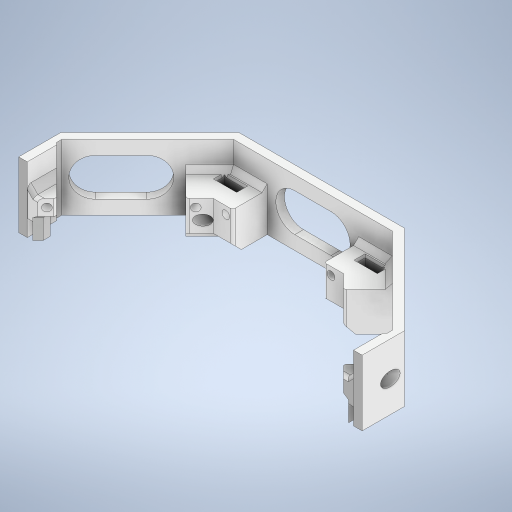
# Autodesk Inventor part: Držák TF-Luna
Saved by Autodesk Inventor 2024 (Build 280153000, 153)
## iProperties
Created: 2023-11-02
Part Number: Držák TF-Luna
Material: Všeobecné
Document SubType Name: Modeling
Designer: 42060
Density: 1 g/cm^3
Appearance: Výchozí
Author: 42060
Autodesk Inventor part; units mm, degrees
ref_plane "YZ Plane" through (0, 0, 0) normal (1, 0, 0) x (0, 1, 0)
ref_plane "XZ Plane" through (0, 0, 0) normal (0, 1, 0) x (-1, 0, 0)
ref_plane "XY Plane" through (0, 0, 0) normal (0, 0, 1) x (1, 0, 0)
sketch "Náčrt1" plane through (0, 0, 0) normal (0, 0, 1) x (1, 0, 0)
  line L0 (0, 0) -> (0, -2.5)
  line L1 (0, -2.5) -> (23, -2.5)
  line L2 (23, -2.5) -> (47.25, -26.75)
  line L3 (49.75, -25.7145) -> (24.0355, 0)
  line L4 (24.0355, 0) -> (0, 0)
  line L5 (49.75, -25.7145) -> (49.75, -37.923)
  line L6 (49.75, -37.923) -> (47.25, -37.923)
  line L7 (47.25, -37.923) -> (47.25, -26.75)
  dimension "d0" = 2.5
  dimension "d1" = 23
  dimension "d2" = 135
  dimension "d50" = 49.75
  dimension "d54" = 2.5
  dimension "d55" = 2.5
  dimension "d156" = 37.923
  constraints: 16 end point, 3 perpendicular, 2 vertical, 1 parallel
  measures "d0" distance of L0.start L0.end
  measures "d1" distance of L0.end L1.end
  measures "d2" angle of L2 L1
  measures "d50" distance between parallel lines of L5 L0
  measures "d54" distance between parallel lines of L2 L3
  measures "d55" distance between parallel lines of L5 L7
  measures "d156" distance between parallel lines of L6 L4
extrude "Vysunutí1" add sketch "Náčrt1" along normal mid plane 19
sketch "Náčrt2" plane through (0, -2.5, 9.5) normal (0, -1, 0) x (1, 0, 0)
  line L0 (23, -19) -> (23, 0) projected
  line L1 (0, 0) -> (23, 0) projected
  line L2 (0, -19) -> (0, 0) projected
  line L3 (23, -19) -> (0, -19) projected
  line L4 (13.25, -7.75) -> (15.25, -7.75)
  arc A0 (15.25, -12.25) -> (15.25, -7.75) centre (15.25, -10) ccw
  line L5 (15.25, -12.25) -> (13.25, -12.25)
  line L6 (13.25, -12.25) -> (13.25, -7.75)
  point P0 (0, -9.5)
  dimension "d6" = 2.25
  dimension "d8" = 9
  dimension "d148" = 13.25
  dimension "d149" = 15.25
  constraints: 6 end point, 2 point on circle, 2 tangent, 1 centre point, 1 horizontal, 1 parallel, 1 perpendicular
  measures "d6" radius of A0
  measures "d8" distance from line of L3 A0.centre
  measures "d148" distance between parallel lines of L6 L2
  measures "d149" distance from line of L2 A0.centre
extrude "Vysunutí2" add sketch "Náčrt2" along normal blind 10 contours L4 A0 L5 L6
sketch "Náčrt4" plane through (47.25, -26.75, 9.5) normal (-0.7071068, -0.7071068, 0) x (-0.7071068, 0.7071068, 0)
  line L0 (24.5447, 7.75) -> (26.5447, 7.75)
  arc A0 (26.5447, 7.75) -> (26.5447, 12.25) centre (26.5447, 10) ccw
  line L1 (26.5447, 12.25) -> (24.5447, 12.25)
  line L2 (24.5447, 12.25) -> (24.5447, 7.75)
  line L3 (0, 19) -> (0, 0) projected
  line L4 (34.2947, 0) -> (0, 0) projected
  line L5 (34.2947, 19) -> (34.2947, 0) projected
  line L6 (0, 19) -> (34.2947, 19) projected
  line L7 (41.189, 12.25) -> (41.189, 7.75) projected
  line L8 (11.2947, 19) -> (11.2947, 0) construction
  line L9 (-1.9553, 12.25) -> (-1.9553, 7.75)
  line L10 (-1.9553, 7.75) -> (-6.4553, 7.75)
  line L11 (-6.4553, 7.75) -> (-6.4553, 12.25)
  line L12 (-6.4553, 12.25) -> (-1.9553, 12.25)
  point P0 (52.3259, 9.5)
  point P1 (28.7947, 10)
  point P2 (-3.9553, 10)
  dimension "d22" = 15.25
  dimension "d33" = 2.25
  dimension "d39" = 5.5
  dimension "d150" = 13.25
  constraints: 16 end point, 4 perpendicular, 3 point on circle, 3 symmetric about line, 2 horizontal, 2 point on line, 2 tangent, 1 centre point, 1 horizontal alignment, 1 parallel, 1 vertical
  measures "d22" distance from line of L8 A0.centre
  measures "d33" radius of A0
  measures "d39" distance from line of L5 point (28.795, 10)
  measures "d150" distance between parallel lines of L8 L2
extrude "Vysunutí3" add sketch "Náčrt4" along normal blind 10 contours L2 L1 A0 L0 | L9 L10 L11 L12
sketch "Náčrt8" plane through (49.75, -37.923, 9.5) normal (1, 0, 0) x (0, 0, -1)
  line L0 (7.75, 8.673) -> (12.25, 8.673) projected
  line L1 (7.75, 6.6084) -> (7.75, 8.673) projected
  line L2 (12.25, 6.6084) -> (7.75, 6.6084) projected
  line L3 (12.25, 8.673) -> (12.25, 6.6084) projected
  line L4 (12.25, 4.5438) -> (7.75, 4.5438) projected
  line L5 (12.25, 6.6084) -> (12.25, 4.5438) projected
  line L6 (12.25, 6.6084) -> (7.75, 6.6084) projected
  line L7 (7.75, 6.6084) -> (7.75, 4.5438) projected
  point P0 (9.5, 37.923)
extrude "Vysunutí7" cut sketch "Náčrt8" along normal through all
sketch "Náčrt10" plane through (13.25, -2.5, 1.75) normal (0, 0, 1) x (1, 0, 0)
  line L0 (2, -10) -> (0, -10) projected
  line L1 (2, -10) -> (4.25, -10) projected
  line L2 (6.568, -10.9602) -> (8.159, -12.5511) projected
  line L3 (9.5732, -13.9654) -> (8.159, -12.5511) projected
  line L4 (4.25, -10) -> (5.6079, -10)
  line L5 (5.6079, -10) -> (6.568, -10.9602)
  circle A0 centre (7.8444, -4.6004) radius 3.5944
  line L6 (4.25, 0) -> (4.25, -10) projected
  line L7 (13.6391, -3.8891) -> (6.568, -10.9602) projected
  line L8 (4.25, -4.6004) -> (2, -4.6004)
  line L9 (2, 0) -> (2, -10) projected
  line L10 (10.3861, -7.1421) -> (11.9771, -8.7331)
  line L11 (15.2301, -5.4801) -> (8.159, -12.5511) projected
  line L12 (5.6079, -10) -> (6.4689, -7.9213) construction
  line L13 (-13.25, 0) -> (9.75, 0) projected
  line L14 (9.75, 0) -> (34, -24.25) projected
  point P0 (-13.25, 2.5)
  dimension "d70" = 112.5
  constraints: 10 end point, 4 point on line, 3 point on circle, 2 horizontal, 2 tangent, 1 centre point, 1 collinear, 1 equal length, 1 perpendicular
  measures "d70" angle of L4 L12
extrude "Vysunutí9" add sketch "Náčrt10" against normal up to surface (4.5 mm away) contours L9 L8 L6 L1 | L6 A0 L7 L5 L4 | L9 L13 L6 L8 | L7 L10 L11 L2 | L7 L14 L11 L10
sketch "Náčrt6" plane through (47.25, -26.75, 9.5) normal (-0.7071068, -0.7071068, 0) x (-0.7071068, 0.7071068, 0)
  arc A0 (11.3919, 8.2595) -> (11.3919, 10.7405) centre (16.5447, 9.5) ccw
  arc A1 (11.1975, 10.7405) -> (11.1975, 8.2595) centre (6.0447, 9.5) ccw
  line L0 (0, 19) -> (0, 0) projected
  line L1 (24.5447, 12.25) -> (24.5447, 7.75) projected
  line L2 (-1.9553, 7.75) -> (-1.9553, 12.25) projected
  line L3 (16.5447, 9.5) -> (24.5447, 9.5) construction
  line L4 (6.0447, 9.5) -> (-1.9553, 9.5) construction
  arc A2 (11.3919, 8.2595) -> (11.1975, 8.2595) centre (11.2947, 8.2361) ccw
  arc A3 (11.1975, 10.7405) -> (11.3919, 10.7405) centre (11.2947, 10.7639) ccw
  arc A4 (11.2947, 7.8606) -> (11.2947, 11.1394) centre (16.5447, 9.5) ccw
  arc A5 (11.2947, 11.1394) -> (11.2947, 7.8606) centre (6.0447, 9.5) ccw
  line L5 (16.5447, 4) -> (6.0447, 4)
  line L6 (16.5447, 15) -> (6.0447, 15)
  point P0 (52.3259, 9.5)
  point P1 (12.5018, 10.2263)
  point P2 (12.5018, 8.7737)
  point P3 (0, 9.5)
  point P4 (12.599, 10.7405)
  point P5 (12.4046, 10.7405)
  point P6 (12.4046, 8.2595)
  point P7 (12.599, 8.2595)
  dimension "d44" = 10.6
  dimension "d45" = 10.5
  dimension "d48" = 0.2
  dimension "d114" = 0.2
  constraints: 16 point on circle, 8 end point, 7 tangent, 6 centre point, 3 point on line, 2 equal radius, 2 horizontal alignment, 1 collinear, 1 midpoint, 1 parallel, 1 perpendicular, 1 other
  measures "d44" diameter of A1
  measures "d45" distance of L4.start L3.start
  measures "d48" diameter of A2
  measures "d114" radial gap between concentric circles of A0 A4
extrude "Vysunutí5" cut sketch "Náčrt6" against normal blind 11.5 contours A2 A1 A3 A0 | A5 A4 | A4 L5 A5 | A4 A5 L6
sketch "Náčrt7" plane through (0, -2.5, 9.5) normal (0, -1, 0) x (1, 0, 0)
  arc A0 (0.0972, -10.7405) -> (0.0972, -8.2595) centre (5.25, -9.5) ccw
  line L0 (0, -19) -> (0, 0) projected
  arc A1 (0, -8.3361) -> (0.0972, -8.2595) centre (0, -8.2361) ccw
  arc A2 (0.0972, -10.7405) -> (0, -10.6639) centre (0, -10.7639) ccw
  arc A3 (-0.0972, -8.2595) -> (-0.0972, -10.7405) centre (-5.25, -9.5) ccw
  arc A4 (-0.0972, -8.2595) -> (0, -8.3361) centre (0, -8.2361) ccw
  arc A5 (0, -10.6639) -> (-0.0972, -10.7405) centre (0, -10.7639) ccw
  arc A6 (0, -7.8606) -> (0, -11.1394) centre (-5.25, -9.5) ccw
  arc A7 (0, -11.1394) -> (0, -7.8606) centre (5.25, -9.5) ccw
  line L1 (-5.25, -4) -> (5.25, -4)
  line L2 (-5.25, -15) -> (5.25, -15)
  point P0 (0, -9.5)
  point P1 (0, -9.5)
  point P2 (0, -8.7737)
  point P3 (0, -10.2263)
  point P4 (0, -9.5)
  point P5 (0.0972, -8.2595)
  point P6 (0, -8.3361)
  point P7 (0, -10.6639)
  point P8 (0.0972, -10.7405)
  point P9 (0, -8.1361)
  point P10 (0, -10.8639)
  point P11 (0, -11.1394)
  point P12 (0, -15)
  point P13 (0, -4)
  dimension "d40" = 10.6
  dimension "d41" = 5.25
  dimension "d49" = 0.2
  dimension "d115" = 0.2
  constraints: 20 point on circle, 8 centre point, 6 tangent, 4 end point, 3 symmetric about line, 2 midpoint, 2 point on line, 2 vertical alignment, 1 equal radius, 1 horizontal alignment, 4 other
  measures "d40" diameter of A0
  measures "d41" distance from line of A0.centre L0
  measures "d49" diameter of A1
  measures "d115" radial gap between concentric circles of A3 A6
extrude "Vysunutí4" cut sketch "Náčrt7" against normal blind 11.5 contours A2 L0 A1 A0 | A0 A1 L0 A7 A2 | A5 A3 A4 L0 | A7 L2 L0 | L0 L1 A7
sketch "Náčrt11" plane through (0, 0, -9.5) normal (0, 0, -1) x (-1, 0, 0)
  line L0 (-23, -2.5) -> (0, -2.5) projected
  line L1 (-47.25, -26.75) -> (-23, -2.5) projected
  line L2 (-13.25, -2.5) -> (-13.25, -12.5) projected
  line L3 (-13.25, -12.5) -> (-18.8579, -12.5) projected
  line L4 (-18.8579, -12.5) -> (-22.8232, -16.4654) projected
  line L5 (-29.8943, -9.3943) -> (-22.8232, -16.4654) projected
  arc A0 (-23.6361, -9.6421) -> (-17.5, -7.1004) centre (-21.0944, -7.1004) ccw projected
  line L6 (-17.5, -7.1004) -> (-17.5, -2.5) projected
  line L7 (-26.8891, -6.3891) -> (-23.6361, -9.6421) projected
  point P0 (0, 0)
extrude "Vysunutí10" add sketch "Náčrt11" against normal up to surface (6.75 mm away) contours L0 L2 L3 L4 L5 L1 L7 A0 L6
sketch "Náčrt3" plane through (0, -12.5, 9.5) normal (0, -1, 0) x (1, 0, 0)
  arc A0 (15.25, -12.25) -> (15.25, -7.75) centre (15.25, -10) ccw projected
  point P0 (0, -9.5)
  constraints: 1 coincident
hole "Díra1" at (15.25, -12.5, -0.5) direction (0, 1, 0) diameter 2.2 end through all
sketch "Náčrt5" plane through (40.1789, -33.8211, 9.5) normal (-0.7071068, -0.7071068, 0) x (0, 0, -1)
  arc A0 (7.75, -26.5447) -> (12.25, -26.5447) centre (10, -26.5447) ccw projected
  line L0 (12.25, 6.4553) -> (7.75, 6.4553) projected
  line L1 (7.75, 6.4553) -> (7.75, 1.9553) projected
  line L2 (7.75, 1.9553) -> (12.25, 1.9553) projected
  line L3 (12.25, 1.9553) -> (12.25, 6.4553) projected
  line L4 (12.25, 1.9553) -> (12.25, 6.4553) projected
  line L5 (12.25, 6.4553) -> (7.75, 6.4553) projected
  line L6 (19, 1.0355) -> (0, 1.0355) projected
  line L7 (0, 9.6683) -> (0, 1.0355) projected
  line L8 (19, 9.6683) -> (0, 9.6683) projected
  line L9 (19, 1.0355) -> (19, 9.6683) projected
  line L10 (19, -11.2947) -> (0, -11.2947) construction
  point P0 (9.5, -52.3259)
  point P1 (10, 3.9553)
  constraints: 1 coincident, 1 symmetric about line
hole "Díra2" at (21.409, -15.0511, -0.5) at (42.9758, -36.6179, -0.5) direction (0.7071068, 0.7071068, 0) diameter 2.2 end through all
chamfer "Zkosení3" [suppressed]
sketch "Náčrt9" plane through (47.25, -35.8792, 1.75) normal (0, 0, 1) x (1, 0, 0)
  line L0 (0, -2.0438) -> (0, 9.1292) projected
  line L1 (0, 0) -> (-2.5065, -2.5065) projected
  line L2 (0, -2.0438) -> (-2.0438, -2.0438)
  line L3 (-2.0438, -2.0438) -> (-2.9691, -2.0438)
  line L4 (-2.5065, -2.5065) -> (-5.6884, 0.6755) projected
  line L5 (0, 9.1292) -> (0, -2.0438) projected
  point P0 (-47.25, 35.8792)
  constraints: 4 end point, 2 horizontal, 2 point on line
extrude "Vysunutí8" add sketch "Náčrt9" against normal up to surface (4.5 mm away) contours L2 L1 L0
extrude "Vysunutí17" cut sketch "Náčrt9" against normal through all contours L1 L4 L3
sketch "Náčrt25" plane through (47.25, -35.8792, -2.75) normal (0, 0, -1) x (-1, 0, 0)
  line L0 (1.5, 2.9562) -> (1.5, -2.0438)
  line L1 (1.5, -2.0438) -> (3, -0.5438)
  line L2 (3, -0.5438) -> (3, 1.4562)
  line L3 (3, 1.4562) -> (1.5, 2.9562)
  line L4 (0, -2.0438) -> (0, 9.1292) projected
  point P0 (47.25, 35.8792)
  dimension "d185" = 45
  dimension "d188" = 1.5
  dimension "d189" = 5
  dimension "d190" = 1.5
  dimension "d191" = 45
  constraints: 8 end point, 1 horizontal alignment, 1 parallel, 1 vertical
  measures "d185" angle of L3 L0
  measures "d188" distance between parallel lines of L0 L2
  measures "d189" distance of L0.start L0.end
  measures "d190" distance between parallel lines of L4 L0
  measures "d191" angle of L0 L1
extrude "Vysunutí24" add sketch "Náčrt25" along normal up to surface (6.75 mm away)
chamfer "Zkosení4" [suppressed]
chamfer "Zkosení10" distance 2 angle 45 2 edges at (47.25, -33.7191, 1.75) (47.25, -33.7191, -2.75)
chamfer "Zkosení11" distance 1.0388 angle 45 3 edges at (44.75, -33.923, -2.75) (44.25, -35.423, -2.75) (44.75, -36.923, -2.75)
sketch "Náčrt26" plane through (47.25, -37.923, 9.5) normal (0, -1, 0) x (1, 0, 0)
  line L0 (0, -14.25) -> (-1.5, -14.25)
  line L1 (2.5, -19) -> (2.5, 0) projected
  line L2 (0, 0) -> (2.5, 0) projected
  line L3 (0, -5.75) -> (0, 0) projected
  line L4 (-2, -7.75) -> (0, -5.75) projected
  line L5 (-2.9691, -7.75) -> (-2, -7.75) projected
  line L6 (-2.9691, -12.25) -> (-2.9691, -7.75) projected
  line L7 (-2.9691, -12.25) -> (-2.9691, -12.25) projected
  line L8 (-2.9691, -12.25) -> (-1.5, -13.2888) projected
  line L9 (-1.5, -12.75) -> (-1.5, -13.2888) projected
  line L10 (0, -14.25) -> (-1.5, -12.75) projected
  line L11 (0, -19) -> (0, -14.25) projected
  line L12 (2.5, -19) -> (0, -19) projected
  line L13 (-1.5, -13.2888) -> (-1.5, -19) projected
  point P0 (-47.25, -9.5)
  constraints: 2 end point, 1 horizontal
extrude "Vysunutí25" add sketch "Náčrt26" against normal up to surface contours L0 L13 L9 L10 surface through (44.25, -34.423, -2.75) normal (-0.7071068, 0.7071068, 0)
extrude "Vysunutí21" add sketch "Náčrt11" against normal blind 2.5 contours L0 L6 A0 L7 L1
sketch "Náčrt22" plane through (17.5, -2.5, -7) normal (0, 0, 1) x (1, 0, 0)
  line L0 (0, -2.4004) -> (5.75, -2.4004)
  line L1 (5.75, -2.4004) -> (5.75, -4.6004)
  line L2 (5.75, -4.6004) -> (0, -4.6004)
  line L3 (0, -4.6004) -> (0, -2.4004)
  line L4 (0, -4.6004) -> (0, 0) projected
  arc A0 (0, -4.6004) -> (6.1361, -7.1421) centre (3.5944, -4.6004) ccw projected
  line L5 (9.3891, -3.8891) -> (6.1361, -7.1421) projected
  line L6 (5.5, 0) -> (9.3891, -3.8891) projected
  line L7 (0, 0) -> (5.5, 0) projected
  point P0 (-17.5, 2.5)
  point P1 (0, -2.4004)
  dimension "d163" = 5.75
  dimension "d164" = 2.2
  constraints: 8 end point, 2 parallel, 1 collinear, 1 horizontal, 1 perpendicular, 1 point on line
  measures "d163" distance of L1.end L2.end
  measures "d164" distance of L0.end L1.end
extrude "Vysunutí20" add sketch "Náčrt22" along normal up to surface (8.75 mm away) contours L4 L7 L6 L5 A0 L2 L1 L0
sketch "Náčrt23" plane through (17.5, -4.9004, -7) normal (0, -1, 0) x (1, 0, 0)
  line L0 (5.75, 8.75) -> (0, 8.75) projected
  line L1 (0, 0) -> (0, 8.75) projected
  line L2 (5.75, 0) -> (0, 0) projected
  line L3 (5.75, 0) -> (5.75, 8.75) projected
  line L4 (0, 1.6599) -> (2.875, 0)
  line L5 (2.875, 0) -> (5.75, 1.6599)
  circle A0 centre (2.875, 3.3198) radius 2.875 construction
  point P0 (-17.5, 7)
  dimension "d169" = 120
  constraints: 4 end point, 3 tangent, 2 point on line, 1 centre point, 1 horizontal alignment, 1 midpoint
  measures "d169" angle of L5 L4
extrude "Vysunutí22" add sketch "Náčrt23" along normal up to surface (2.2 mm away) contours L3 L2 L5 | L4 L2 L1
hole "Díra6" at (20.375, -4.9004, -3.6802) direction (0, 1, 0) diameter 3 end through all both
sketch "Náčrt24" plane through (0, 0, -9.5) normal (0, 0, -1) x (-1, 0, 0)
  line L0 (0, 0) -> (-24.0355, 0) projected
  line L1 (-17.5, -7.1004) -> (-17.5, -4.9004) projected
  line L2 (-17.5, -7.1004) -> (-17.5, -4.9004) projected
  line L3 (-21.875, 0) -> (-18.875, 0) projected
  line L4 (-18.875, -4.9004) -> (-21.875, -4.9004) projected
  line L5 (-23.25, -2) -> (-17.5, -2)
  line L6 (-23.25, -2) -> (-22.7141, 0)
  line L7 (-17.5, -2) -> (-18.0359, 0)
  point P0 (-20.375, -2)
  point P1 (-20.375, -4.9004)
  dimension "d180" = 2
  dimension "d183" = 75
  dimension "d184" = 75
  constraints: 6 end point, 3 point on line, 2 midpoint, 1 vertical alignment
  measures "d180" distance between parallel lines of L0 L5
  measures "d183" angle of L0 L6
  measures "d184" angle of L0 L7
extrude "Vysunutí23" cut sketch "Náčrt24" against normal blind 10
fillet "Zaoblení1" radius 1 2 edges at (46.25, -37.923, 2.75) (44.7654, -37.923, 1.75)
chamfer "Zkosení5" distance 1.5 angle 45 2 edges at (26.4471, -5.9471, 1.75) (18.125, -2.5, 1.75)
sketch "Náčrt12" plane through (0, 0, 9.5) normal (0, 1, 0) x (1, 0, 0)
  circle A0 centre (15.25, 10) radius 1.1 projected
  line L0 (15.25, 12.4249) -> (17.35, 11.2124)
  line L1 (17.35, 11.2124) -> (17.35, 8.7876)
  line L2 (17.35, 8.7876) -> (15.25, 7.5751)
  line L3 (15.25, 7.5751) -> (13.15, 8.7876)
  line L4 (13.15, 8.7876) -> (13.15, 11.2124)
  line L5 (13.15, 11.2124) -> (15.25, 12.4249)
  point P0 (0, 9.5)
  point P1 (15.25, 10)
  dimension "d81" = 4.2
  constraints: 12 end point, 1 coincident, 1 vertical alignment, 13 other
  measures "d81" distance between parallel lines of L4 L1
extrude "Vysunutí12" [suppressed]
sketch "Náčrt13" plane through (24.0355, 0, -9.5) normal (0.7071068, 0.7071068, 0) x (-0.7071068, 0.7071068, 0)
  circle A0 centre (-8.7855, 9) radius 1.1 projected
  line L0 (-8.7855, 6.5751) -> (-10.8855, 7.7876)
  line L1 (-10.8855, 7.7876) -> (-10.8855, 10.2124)
  line L2 (-10.8855, 10.2124) -> (-8.7855, 11.4249)
  line L3 (-8.7855, 11.4249) -> (-6.6855, 10.2124)
  line L4 (-6.6855, 10.2124) -> (-6.6855, 7.7876)
  line L5 (-6.6855, 7.7876) -> (-8.7855, 6.5751)
  line L6 (-39.2855, 6.5751) -> (-41.3855, 7.7876)
  line L7 (-41.3855, 7.7876) -> (-41.3855, 10.2124)
  line L8 (-41.3855, 10.2124) -> (-39.2855, 11.4249)
  line L9 (-39.2855, 11.4249) -> (-37.1855, 10.2124)
  line L10 (-37.1855, 10.2124) -> (-37.1855, 7.7876)
  line L11 (-37.1855, 7.7876) -> (-39.2855, 6.5751)
  circle A1 centre (-39.2855, 9) radius 1.1 projected
  point P0 (16.9957, 9.5)
  point P1 (-39.2855, 9)
  point P2 (-39.2855, 9)
  dimension "d84" = 4.2
  dimension "d85" = 4.2
  constraints: 24 end point, 3 coincident, 1 vertical alignment, 26 other
  measures "d84" distance between parallel lines of L4 L1
  measures "d85" distance between parallel lines of L7 L10
extrude "Vysunutí13" [suppressed]
extrude "Vysunutí14" [suppressed]
sketch "Náčrt15" plane through (0, 0, 9.5) normal (0, 1, 0) x (1, 0, 0)
  circle A0 centre (15.25, 10) radius 1.1 projected
  point P0 (0, 9.5)
  point P1 (15.25, 10)
  constraints: 1 coincident
hole "Díra3" at (15.25, 0, -0.5) direction (0, -1, 0) diameter 4 depth 2
sketch "Náčrt16" plane through (24.0355, 0, -9.5) normal (0.7071068, 0.7071068, 0) x (-0.7071068, 0.7071068, 0)
  circle A0 centre (-8.7855, 9) radius 1.1 projected
  point P0 (16.9957, 9.5)
  constraints: 1 coincident
hole "Díra4" at (30.2478, -6.2123, -0.5) direction (-0.7071068, -0.7071068, 0) diameter 4 depth 2
sketch "Náčrt17" plane through (24.0355, 0, -9.5) normal (0.7071068, 0.7071068, 0) x (-0.7071068, 0.7071068, 0)
  circle A0 centre (-39.2855, 9) radius 1.1 projected
  point P0 (16.9957, 9.5)
  point P1 (-39.2855, 9)
  point P2 (-39.2855, 9)
  constraints: 2 coincident
hole "Díra5" at (51.8146, -27.7791, -0.5) direction (-0.7071068, -0.7071068, 0) diameter 4 depth 6
sketch "Náčrt14" plane through (49.75, -37.923, 9.5) normal (1, 0, 0) x (0, 0, -1)
  line L0 (19, 12.2085) -> (0, 12.2085) projected
  line L1 (19, 12.2085) -> (23, 12.2085)
  line L2 (23, 12.2085) -> (23, 6.2085)
  line L3 (23, 6.2085) -> (21, 6.2085)
  line L4 (21, 6.2085) -> (21, 10.2085)
  line L5 (21, 10.2085) -> (19, 10.2085)
  line L6 (19, 12.2085) -> (19, 0) projected
  point P0 (9.5, 37.923)
  point P1 (11.3812, 11.7085)
  dimension "d105" = 2
  dimension "d106" = 2
  dimension "d107" = 6
  dimension "d108" = 4
  constraints: 10 end point, 3 perpendicular, 1 horizontal, 1 vertical, 1 other
  measures "d105" distance between parallel lines of L1 L5
  measures "d106" distance between parallel lines of L4 L2
  measures "d107" distance between parallel lines of L1 L3
  measures "d108" distance between parallel lines of L6 L2
extrude "Vysunutí15" [suppressed]
chamfer "Zkosení7" [suppressed]
chamfer "Zkosení1" distance 2.5 angle 45 2 edges at (16.0539, -12.5, -9.5) (20.8405, -14.4827, -9.5)
fillet "Zaoblení3" radius 0.7 3 edges at (13.25, -12.5, -2.625) (22.8232, -16.4654, -2.625) (41.5616, -35.2037, -0.5)
sketch "Náčrt19" plane through (49.75, -37.923, 9.5) normal (1, 0, 0) x (0, 0, -1)
  line L0 (0, 11.173) -> (0, 0) projected
  line L1 (0, 0) -> (19, 0)
  line L2 (19, 0) -> (19, -0.077)
  line L3 (19, -0.077) -> (0, -0.077)
  line L4 (0, -0.077) -> (0, 0)
  point P0 (9.5, 37.923)
  dimension "d153" = 38
  constraints: 8 end point, 2 parallel, 1 horizontal, 1 perpendicular
  measures "d153" distance from line of point (9.5, 37.923) L3
extrude "Vysunutí18" add sketch "Náčrt19" against normal up to surface (2.5 mm away)
sketch "Náčrt20" plane through (0, 0, 9.5) normal (0, 0, 1) x (1, 0, 0)
  line L0 (23, -2.5) -> (47.25, -26.75) projected
  line L1 (47.25, -26.75) -> (48.6326, -28.1326)
  line L2 (48.6326, -28.1326) -> (47.25, -29.5152)
  line L3 (47.25, -26.75) -> (47.25, -38) projected
  line L4 (47.8826, -27.3826) -> (47.8826, -28.8826)
  line L5 (45.25, -31.5152) -> (42.0565, -34.7087) projected
  point P0 (0, 0)
  dimension "d159" = 0.75
  constraints: 6 end point, 4 point on line, 1 collinear, 1 perpendicular, 1 vertical
  measures "d159" distance from line of L1.end L4
extrude "Vysunutí19" cut sketch "Náčrt20" against normal through all contours L1 L4 L2 L3
chamfer "Zkosení12" distance 0.75 angle 45 1 edges at (46.5, -32.173, -4)
chamfer "Zkosení13" distance 0.5 angle 45 4 edges at (17.5, -6.0004, 1.75) (20.375, -7.1004, 1.75) (20.375, -4.9004, 1.75) (23.25, -6.0004, 1.75)
mirror "Zrcadlit1" about plane through (0, 0, 0) normal (1, 0, 0)
